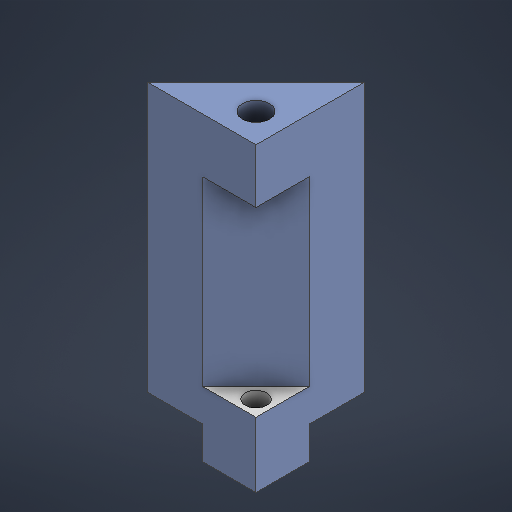
# Autodesk Inventor part: bracket servo
Saved by Autodesk Inventor 2025.1 (Build 291241000, 241)
## iProperties
Created: 2025-01-24
Part Number: bracket servo
Material: Generic
Document SubType Name: Modeling
Designer: m_kni
Density: 1 g/cm^3
Appearance: Default
Finish1_Area: 954.216 mm^2
Finish1_Appearance: Rubber - Blue
Finish1_Process: Prime/Paint RAL 3018
Finish1_Description: Prime/Paint RAL 3018
Finish1_ShortDescription: RAL 3018
Finish1_Thickness: 0.050 mm
Author: m_kni
## iProperties of the stored document bracket servo_3DPrint.ipt
Created: 2025-01-30
Part Number: bracket servo_3DPrint
Material: Generic
Document SubType Name: Modeling
Designer: m_kni
Density: 1 g/cm^3
Appearance: Default
Author: m_kni
Autodesk Inventor part; units mm, degrees
ref_plane "YZ Plane" through (0, 0, 0) normal (1, 0, 0) x (0, 1, 0)
ref_plane "XZ Plane" through (0, 0, 0) normal (0, 1, 0) x (-1, 0, 0)
ref_plane "XY Plane" through (0, 0, 0) normal (0, 0, 1) x (1, 0, 0)
sketch "Sketch1" plane through (0, 0, 0) normal (0, 1, 0) x (-1, 0, 0)
  line L0 (0, 0) -> (4.95, 0)
  line L1 (0, 0) -> (0, -4.95)
  line L2 (0, -4.95) -> (4.95, 0)
  dimension "d0" = 4.95
  dimension "d1" = 4.95
  constraints: 6 end point, 1 horizontal, 1 vertical
  measures "d0" distance of L0.start L0.end
  measures "d1" distance of L0.start L1.end
extrude "Extrusion1" add sketch "Sketch1" along normal blind 6
sketch "Sketch2" plane through (0, 6, 0) normal (0, 1, 0) x (1, 0, 0)
  line L0 (-4.95, 0) -> (0, 0) projected
  line L1 (0, 0) -> (-10, 0)
  line L2 (0, 0) -> (0, 10)
  line L3 (0, 10) -> (-10, 0)
  dimension "d4" = 10
  dimension "d5" = 10
  constraints: 6 end point, 1 collinear, 1 vertical
  measures "d4" distance of L0.end L1.end
  measures "d5" distance of L0.end L2.end
extrude "Extrusion2" add sketch "Sketch2" along normal blind 2
sketch "Sketch3" plane through (0, 8, 0) normal (0, 1, 0) x (1, 0, 0)
  line L0 (-10, 0) -> (-4.95, 0) projected
  line L1 (-10, 0) -> (-4.95, 0)
  line L2 (0, 4.95) -> (0, 10) projected
  line L3 (-4.95, 0) -> (0, 4.95)
  line L4 (0, 4.95) -> (0, 10)
  line L5 (0, 10) -> (-10, 0)
  point P0 (0, 0)
  constraints: 8 end point, 2 collinear, 1 parallel
extrude "Extrusion3" add sketch "Sketch3" along normal blind 19.75
sketch "Sketch4" plane through (0, 27.75, 0) normal (0, 1, 0) x (1, 0, 0)
  line L0 (-4.95, 0) -> (0, 0) projected
  line L1 (-4.95, 0) -> (0, 0)
  line L2 (-4.95, 0) -> (0, 4.95) projected
  line L3 (0, 0) -> (0, 4.95) projected
  constraints: 2 end point, 1 collinear
extrude "Extrusion4" add sketch "Sketch4" against normal blind 5
sketch "Sketch6" plane through (0, 27.75, 0) normal (0, 1, 0) x (1, 0, 0)
  line L0 (-10, 0) -> (-4.95, 0) projected
  line L1 (-10, 0) -> (0, 10)
  line L2 (0, 10) -> (-10, 0) projected
  line L3 (-4.95, 0) -> (0, 0) projected
  line L4 (0, 0) -> (0, 10) projected
  circle A0 centre (-2.6665, 2.6666) radius 1.25
  dimension "d12" = 2.5
  dimension "d17" = 3.3
  dimension "d18" = 2.6665
  dimension "d19" = 2.6666
  constraints: 2 end point, 1 centre point, 1 collinear
  measures "d12" diameter of A0
  measures "d17" distance from line of A0.centre L1
  measures "d18" distance from line of L4 A0.centre
  measures "d19" distance from line of L3 A0.centre
extrude "Extrusion5" cut sketch "Sketch6" against normal blind 5 contours A0
sketch "Sketch7" plane through (0, 8, 0) normal (0, 1, 0) x (1, 0, 0)
  line L0 (0, 4.95) -> (-4.95, 0) projected
  line L1 (0, 4.95) -> (-4.95, 0)
  line L2 (0, 4.95) -> (-4.95, 0) projected
  line L3 (0, 0) -> (0, 4.95) projected
  line L4 (-4.95, 0) -> (0, 0)
  line L5 (0, 0) -> (0, 4.95)
  constraints: 6 end point, 1 horizontal, 1 perpendicular
extrude "Extrusion6" add sketch "Sketch7" along normal blind 2
sketch "Sketch8" plane through (0, 0, 0) normal (0, -1, 0) x (1, 0, 0)
  line L0 (-4.95, 0) -> (0, 0) projected
  line L1 (0, 0) -> (0, -4.95) projected
  circle A0 centre (-1.45, -1.45) radius 1
  dimension "d20" = 1.45
  dimension "d21" = 1.45
  dimension "d22" = 2
  constraints: 1 centre point, 1 coincident
  measures "d20" distance from line of point (-1.45, -1.45) L0
  measures "d21" distance from line of L1 point (-1.45, -1.45)
  measures "d22" diameter of A0
extrude "Extrusion7" cut sketch "Sketch8" against normal up to surface (10 mm away)
sketch "Sketch9" plane through (0, 27.75, 0) normal (0, 1, 0) x (1, 0, 0)
  line L0 (0, 10) -> (10.5977, -0.5977)
  line L1 (0, 0) -> (0, 10) projected
  line L2 (0, 10) -> (-10, 0) projected
  line L3 (0, 10) -> (11.6673, -1.6673)
  line L4 (11.6673, -1.6673) -> (1.6673, -11.6673)
  line L5 (11.6673, -1.6673) -> (30.5491, -1.6673) construction
  line L6 (-10, 0) -> (1.6673, -11.6673)
  arc A0 (8.435, -4.8995) -> (4.8995, -8.435) centre (6.6673, -6.6673) ccw
  line L7 (6.6673, -6.6673) -> (4.8995, -4.8995)
  circle A1 centre (4.8995, -4.8995) radius 1.25
  dimension "d25" = 45
  dimension "d26" = 16.5
  dimension "d27" = 135
  dimension "d28" = 5
  dimension "d29" = 2.5
  constraints: 12 end point, 3 point on circle, 3 point on line, 2 centre point, 2 coincident, 1 horizontal, 1 midpoint, 1 perpendicular
  measures "d25" angle of L1 L0
  measures "d26" distance of L0.start L3.end
  measures "d27" angle of L4 L5
  measures "d28" diameter of A0
  measures "d29" diameter of A1
sketch "Sketch10" plane through (0, 10, 0) normal (0, 1, 0) x (1, 0, 0)
  line L0 (-4.95, 0) -> (0, 0) projected
  line L1 (-4.95, 0) -> (0, 4.95) projected
  line L2 (0, 0) -> (0, 4.95) projected
  circle A0 centre (-1.45, 1.45) radius 1 projected
  circle A1 centre (-1.45, 1.45) radius 1 projected
  line L3 (0, 0) -> (0, 4.95) projected
  line L4 (-4.95, 0) -> (0, 4.95) projected
  line L5 (-4.95, 0) -> (0, 0) projected
extrude "Extrusion8" cut sketch "Sketch10" against normal blind 4
sketch "Sketch11" plane through (0, 6, 0) normal (0, -1, 0) x (1, 0, 0)
  line L0 (-3.3378, -1.6122) -> (-4.95, 0) projected
  line L1 (-1.6121, -3.3379) -> (-3.3378, -1.6122) projected
  line L2 (0, -4.95) -> (-1.6121, -3.3379) projected
  line L3 (0, -4.95) -> (0, 0) projected
  line L4 (0, 0) -> (0, -10) projected
  line L5 (0, -4.95) -> (0, -10) projected
  line L6 (-10, 0) -> (-4.95, 0) projected
  line L7 (-10, 0) -> (0, 0) projected
  line L8 (0, 0) -> (-4.95, 0) projected
  circle A0 centre (-1.45, -1.45) radius 1 projected
  line L9 (0, -4.95) -> (0, 0) projected
  line L10 (0, 0) -> (-4.95, 0) projected
  line L11 (0, -4.95) -> (-4.95, 0) projected
  line L12 (0, -4.95) -> (-1.6121, -3.3379) projected
  line L13 (-1.6121, -3.3379) -> (-3.3378, -1.6122) projected
  line L14 (-3.3378, -1.6122) -> (-4.95, 0) projected
  line L15 (0, -4.95) -> (-4.95, 0) projected
  line L16 (0, -4.95) -> (0, -10) projected
  line L17 (0, 0) -> (0, -10) projected
  line L18 (0, -4.95) -> (0, 0) projected
  line L19 (0, 0) -> (-4.95, 0) projected
  line L20 (-10, 0) -> (0, 0) projected
  line L21 (-10, 0) -> (-4.95, 0) projected
  line L22 (0, -4.95) -> (-4.95, 0) projected
  line L23 (0, 0) -> (-4.95, 0) projected
  line L24 (0, -4.95) -> (0, 0) projected
  circle A1 centre (-1.45, -1.45) radius 1 projected
  line L25 (0, -10) -> (-10, 0) projected
  line L26 (0, -10) -> (-10, 0) projected
  arc A2 (-1.6121, -3.3379) -> (-3.3378, -1.6122) centre (-2.6665, -2.6666) ccw projected
  arc A3 (-3.3378, -1.6122) -> (-1.6121, -3.3379) centre (-2.6665, -2.6666) ccw projected
  line L27 (-1.6121, -3.3379) -> (-3.3378, -1.6122) projected
  arc A4 (-3.3378, -1.6122) -> (-1.6121, -3.3379) centre (-2.6665, -2.6666) ccw projected
  circle A5 centre (-2.6665, -2.6666) radius 1.25 projected
  arc A6 (-1.6121, -3.3379) -> (-3.3378, -1.6122) centre (-2.6665, -2.6666) ccw projected
  arc A7 (-3.3378, -1.6122) -> (-1.6121, -3.3379) centre (-2.6665, -2.6666) ccw projected
  circle A8 centre (-2.6665, -2.6666) radius 1.25 projected
  line L28 (0, -10) -> (-10, 0) projected
  circle A9 centre (-2.6665, -2.6666) radius 1.25 projected
  line L29 (0, 0) -> (0, -10) projected
  line L30 (0, -10) -> (-10, 0) projected
  line L31 (-10, 0) -> (0, 0) projected
  arc A10 (-1.6121, -3.3379) -> (-3.3378, -1.6122) centre (-2.6665, -2.6666) ccw projected
  line L32 (0, -4.95) -> (-1.6121, -3.3379) projected
  line L33 (0, -4.95) -> (0, 0) projected
  line L34 (0, 0) -> (-4.95, 0) projected
  line L35 (-3.3378, -1.6122) -> (-4.95, 0) projected
  line L36 (0, -4.95) -> (-4.95, 0) projected
  circle A11 centre (-1.45, -1.45) radius 1 projected
  line L37 (0, 0) -> (0, -4.95) projected
  line L38 (-4.95, 0) -> (0, 0) projected
  line L39 (0, -4.95) -> (-4.95, 0) projected
  line L40 (0, -4.95) -> (-4.95, 0) projected
  circle A12 centre (-1.45, -1.45) radius 1 projected
  circle A13 centre (-1.45, -1.45) radius 1 projected
  line L41 (0, -4.95) -> (0, 0) projected
  line L42 (0, 0) -> (0, -4.95) projected
  line L43 (0, 0) -> (-4.95, 0) projected
  line L44 (-4.95, 0) -> (0, 0) projected
  circle A14 centre (-1.45, -1.45) radius 1 projected
  line L45 (-4.95, 0) -> (0, 0) projected
  line L46 (0, -4.95) -> (-4.95, 0) projected
  line L47 (0, 0) -> (0, -4.95) projected
  line L48 (0, -4.95) -> (-4.95, 0) projected
  line L49 (-10, 0) -> (-4.95, 0) projected
  line L50 (0, -10) -> (-10, 0) projected
  line L51 (0, -4.95) -> (0, -10) projected
  line L52 (0, -10) -> (-10, 0) projected
  line L53 (0, 0) -> (0, -10) projected
  line L54 (0, -10) -> (-10, 0) projected
  line L55 (-3.3378, -1.6122) -> (-1.6121, -3.3379)
  constraints: 2 end point, 1 collinear, 7 other
extrude "Extrusion9" add sketch "Sketch11" along normal blind 3 contours A3 L2 L4 L25 L6 L0 | L1 A3
body "Solid1"
